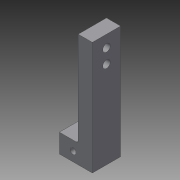
# Autodesk Inventor part: X_Rail_Belt_Pulley_Connector
Saved by Autodesk Inventor 2015 (Build 190159000, 159)
## iProperties
Created: 2017-02-16
Part Number: X_Rail_Belt_Pulley_Connector
Material: Generic
Document SubType Name: Modeling
Designer: Guy
Density: 1 g/cm^3
Appearance: Default
Mass: 41.0677 g
Surface Area: 102.64 cm^2
Volume: 41.0677 cm^3
Author: Guy
Autodesk Inventor part; units mm, degrees
ref_plane "YZ Plane" through (0, 0, 0) normal (1, 0, 0) x (0, 1, 0)
ref_plane "XZ Plane" through (0, 0, 0) normal (0, 1, 0) x (-1, 0, 0)
ref_plane "XY Plane" through (0, 0, 0) normal (0, 0, 1) x (1, 0, 0)
sketch "Sketch1" plane through (0, 0, 0) normal (0, 0, 1) x (1, 0, 0)
  line L0 (0, 0) -> (35, 0)
  line L1 (35, 0) -> (35, 30)
  line L2 (35, 30) -> (0, 30)
  line L3 (0, 30) -> (0, 0)
  dimension "d0" = 35
  dimension "d1" = 30
  constraints: 8 end point, 2 parallel, 1 horizontal, 1 perpendicular
  measures "d0" distance of L1.end L2.end
  measures "d1" distance of L0.end L1.end
extrude "Extrusion1" add sketch "Sketch1" along normal blind 110
sketch "Sketch2" plane through (0, 0, 110) normal (0, 0, 1) x (1, 0, 0)
  line L0 (0, 0) -> (35, 0) projected
  line L1 (35, 0) -> (35, 30) projected
  line L2 (35, 30) -> (0, 30) projected
  line L3 (0, 30) -> (0, 0) projected
  line L4 (0, 0) -> (35, 0) projected
  line L5 (35, 30) -> (20, 30)
  line L6 (20, 30) -> (20, 0)
  line L7 (20, 0) -> (35, 0)
  line L8 (35, 0) -> (35, 30)
  dimension "d4" = 15
  constraints: 8 end point, 2 parallel, 1 horizontal, 1 perpendicular, 1 point on line
  measures "d4" distance between parallel lines of L6 L1
extrude "Extrusion2" cut sketch "Sketch2" against normal blind 90 contours L3 L2 L6 L0
sketch "Sketch3" plane through (35, 0, 0) normal (1, 0, 0) x (0, 0, -1)
  line L0 (0, 0) -> (0, 30) projected
  line L1 (0, 30) -> (-110, 30) projected
  line L2 (-110, 0) -> (-110, 30) projected
  line L3 (0, 0) -> (-110, 0) projected
  circle A0 centre (-97.5, 15) radius 4
  circle A1 centre (-82.5, 15) radius 4
  point P0 (0, 0)
  dimension "d9" = 15
  dimension "d10" = 15
  dimension "d11" = 12.5
  dimension "d12" = 15
  dimension "d13" = 8
  dimension "d14" = 8
  constraints: 2 centre point
  measures "d9" distance from line of A0.centre L1
  measures "d10" distance from line of A1.centre L1
  measures "d11" distance from line of A0.centre L2
  measures "d12" distance of A0.centre A1.centre
  measures "d13" diameter of A0
  measures "d14" diameter of A1
extrude "Extrusion3" cut sketch "Sketch3" against normal up to next contours A0 | A1
sketch "Sketch4" plane through (0, 30, 0) normal (0, 1, 0) x (1, 0, 0)
  circle A0 centre (14.5, -10) radius 3.175
  line L0 (0, 0) -> (0, -20) projected
  line L1 (0, -20) -> (20, -20) projected
  line L2 (35, 0) -> (0, 0) projected
  dimension "d17" = 6.35
  dimension "d18" = 14.5
  dimension "d23" = 10
  constraints: 1 centre point
  measures "d17" diameter of A0
  measures "d18" distance from line of L0 A0.centre
  measures "d23" distance from line of L2 A0.centre
extrude "Extrusion4" cut sketch "Sketch4" against normal up to next
fillet "Fillet1" radius 2 1 edges at (20, 15, 20)
body "Solid1"
